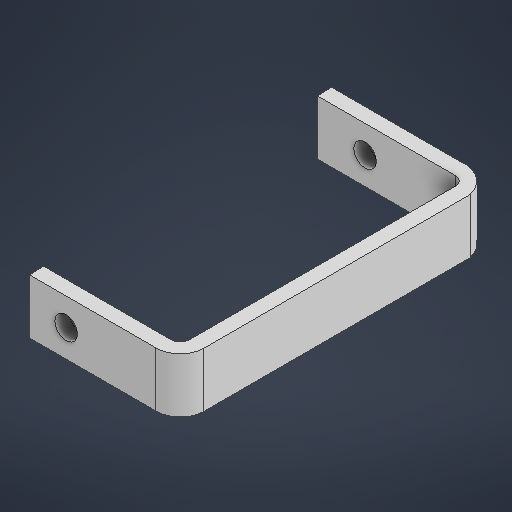
# Autodesk Inventor part: Side bar holding bracket
Saved by Autodesk Inventor 2027 (Build 310192000, 192)
## iProperties
Created: 2026-04-16
Part Number: Side bar holding bracket
Material: Generic
Document SubType Name: Modeling
Designer: ratik
Density: 1 g/cm^3
Appearance: Default
Author: ratik
Autodesk Inventor part; units mm, degrees
ref_plane "YZ Plane" through (0, 0, 0) normal (1, 0, 0) x (0, 1, 0)
ref_plane "XZ Plane" through (0, 0, 0) normal (0, 1, 0) x (-1, 0, 0)
ref_plane "XY Plane" through (0, 0, 0) normal (0, 0, 1) x (1, 0, 0)
sketch "Sketch1" plane through (0, 0, 0) normal (0, 1, 0) x (-1, 0, 0)
  line L0 (20.5369, -73.7451) -> (-17.2994, -73.7451)
  line L1 (-14.2617, -77.74) -> (20.7383, -77.74)
  line L2 (20.7383, -77.74) -> (20.5369, -73.7451)
  line L3 (17.5042, 8.2501) -> (-17.003, 8.2501)
  line L4 (-17.2994, 4.2549) -> (17.7006, 4.2549)
  line L5 (17.7006, 4.2549) -> (17.5042, 8.2501)
  line L6 (-23.7994, -71.2451) -> (-23.7994, 1.7549)
  line L7 (-19.7994, 1.7549) -> (-19.7994, -71.2451)
  arc A0 (-17.2994, 4.2549) -> (-19.7994, 1.7549) centre (-17.2994, 1.7549) ccw
  arc A1 (-17.003, 8.2501) -> (-23.7994, 1.7549) centre (-17.2994, 1.7569) ccw
  arc A2 (-19.7994, -71.2451) -> (-17.2994, -73.7451) centre (-17.2994, -71.2451) ccw
  arc A3 (-23.7994, -71.2451) -> (-14.2617, -77.74) centre (-15.5172, -69.3332) ccw
  point P0 (0, 0)
  dimension "d2" = 4
  dimension "d3" = 4
  dimension "d4" = 35
  dimension "d5" = 35
  dimension "d29" = 78
  dimension "d31" = 73
  dimension "d33" = 2.5
  dimension "d34" = 2.5
  dimension "d36" = 2.5
  dimension "d37" = 4
  dimension "d38" = 6.5
  dimension "d39" = 2.5
  dimension "d41" = 8.5
  constraints: 16 end point, 8 point on circle, 4 centre point, 3 parallel, 2 horizontal
  measures "d2" distance of L1.end L0.start
  measures "d3" distance of L4.end L3.start
  measures "d4" distance of L4.start L4.end
  measures "d5" distance of L1.start L1.end
  measures "d29" distance between parallel lines of L0 L4
  measures "d31" distance of L6.start L6.end
  measures "d33" distance from line of L0.end L7
  measures "d34" distance from line of L7 L4.start
  measures "d36" radius of A0
  measures "d37" distance between parallel lines of L6 L7
  measures "d38" radius of A1
  measures "d39" radius of A2
  measures "d41" radius of A3
extrude "Extrusion1" add sketch "Sketch1" along normal blind 15
sketch "Sketch2" plane through (-17.5042, 0, 8.2501) normal (0, 0, 1) x (1, 0, 0)
  circle A0 centre (10, 7.5) radius 3.1
  line L0 (0, 15) -> (34.5072, 15) projected
  line L1 (0, 0) -> (0, 15) projected
  point P0 (17.5042, 0)
  dimension "d19" = 6.2
  dimension "d20" = 7.5
  dimension "d21" = 10
  constraints: 1 centre point
  measures "d19" diameter of A0
  measures "d20" distance from line of L0 A0.centre
  measures "d21" distance from line of L1 A0.centre
extrude "Extrusion2" cut sketch "Sketch2" against normal blind 120
sketch "Sketch3" plane through (12.7652, 0, -83.1298) normal (-1, 0, 0) x (0, 0, 1)
  circle A0 centre (45, 7.5) radius 3.1
  line L0 (0, 15) -> (90, 15) projected
  line L1 (-6.5, 0) -> (-6.5, 15) projected
  point P0 (83.1298, 0)
  dimension "d24" = 6.2
  dimension "d25" = 7.5
  dimension "d26" = 51.5
  constraints: 1 centre point
  measures "d24" diameter of A0
  measures "d25" distance from line of L0 A0.centre
  measures "d26" distance from line of L1 A0.centre
extrude "Extrusion3" [suppressed]
body "Solid1"
